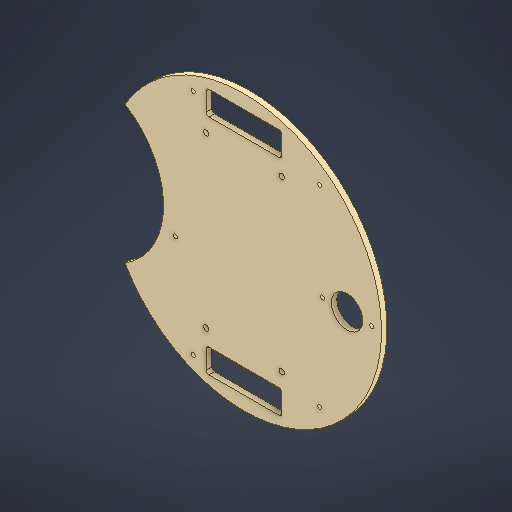
# Autodesk Inventor part: base plate
Saved by Autodesk Inventor 2026.1 (Build 301233000, 233)
## iProperties
Created: 2025-03-16
Part Number: base plate
Material: Generisch
Document SubType Name: Modeling
Designer: sfz
Density: 1 g/cm^3
Appearance: Beige
Author: sfz
Autodesk Inventor part; units mm, degrees
ref_plane "YZ Plane" through (0, 0, 0) normal (1, 0, 0) x (0, 1, 0)
ref_plane "XZ Plane" through (0, 0, 0) normal (0, 1, 0) x (-1, 0, 0)
ref_plane "XY Plane" through (0, 0, 0) normal (0, 0, 1) x (1, 0, 0)
sketch "Skizze1" plane through (0, 0, 0) normal (0, 1, 0) x (-1, 0, 0)
  arc A0 (86.6025, 50) -> (86.6025, -50) centre (0, 0) ccw
  arc A1 (86.6025, 50) -> (86.6025, -50) centre (117.2454, 0) ccw
  line L0 (27.5, 90) -> (-27.5, 90)
  line L1 (-27.5, 90) -> (-27.5, 72.5)
  line L2 (-27.5, 72.5) -> (27.5, 72.5)
  line L3 (27.5, 72.5) -> (27.5, 90)
  line L4 (27.5, -72.5) -> (-27.5, -72.5)
  line L5 (-27.5, -72.5) -> (-27.5, -90)
  line L6 (-27.5, -90) -> (27.5, -90)
  line L7 (27.5, -90) -> (27.5, -72.5)
  circle A2 centre (91, 0) radius 32
  circle A3 centre (27.5, 61.5) radius 2
  circle A4 centre (-27.5, 61.5) radius 2
  circle A5 centre (27.5, -61.5) radius 2
  circle A6 centre (-27.5, -61.5) radius 2
  circle A7 centre (-75, 0) radius 11.5
  circle A8 centre (-57, 0) radius 1.5
  circle A9 centre (-93, 0) radius 1.5
  circle A10 centre (50, -15) radius 1.5
  circle A11 centre (37, -83) radius 1.5
  circle A12 centre (37, 83) radius 1.5
  circle A13 centre (-55, 70) radius 1.5
  circle A14 centre (-55, -70) radius 1.5
  point P0 (58.6025, 0)
  point P1 (27.5, -81.25)
  dimension "d0" = 100
  dimension "d1" = 100
  dimension "d2" = 17.5
  dimension "d3" = 28
  dimension "d4" = 55
  dimension "d5" = 17.5
  dimension "d7" = 72.5
  dimension "d8" = 72.5
  dimension "d9" = 27.5
  dimension "d12" = 64
  dimension "d13" = 4
  dimension "d14" = 4
  dimension "d15" = 4
  dimension "d16" = 4
  dimension "d19" = 11
  dimension "d23" = 11
  dimension "d25" = 27.5
  dimension "d26" = 27.5
  dimension "d43" = 23
  dimension "d48" = 75
  dimension "d49" = 3
  dimension "d50" = 3
  dimension "d51" = 36
  dimension "d52" = 18
  dimension "d95" = 3
  dimension "d96" = 3
  dimension "d97" = 3
  dimension "d98" = 3
  dimension "d99" = 3
  dimension "d100" = 70
  dimension "d101" = 70
  dimension "d102" = 55
  dimension "d103" = 83
  dimension "d104" = 83
  dimension "d105" = 37
  dimension "d106" = 50
  dimension "d108" = 15
  constraints: 16 end point, 15 centre point, 6 horizontal alignment, 5 point on circle, 4 parallel, 4 vertical alignment, 2 horizontal, 2 perpendicular, 2 point on line, 1 coincident, 1 midpoint
  measures "d0" radius of A0
  measures "d1" distance of A1.start A1.end
  measures "d2" distance of L7.start L7.end
  measures "d3" horizontal distance of point (58.603, 0) A1.end
  measures "d4" distance from line of L5 point (27.5, -81.25)
  measures "d5" distance between parallel lines of L2 L0
  measures "d7" distance from line of L2 A0.centre
  measures "d8" distance from line of A0.centre L4
  measures "d9" distance from line of A0.centre L1
  measures "d12" diameter of A2
  measures "d13" diameter of A6
  measures "d14" diameter of A5
  measures "d15" diameter of A3
  measures "d16" diameter of A4
  measures "d19" distance from line of L4 A5.centre
  measures "d23" distance from line of L2 A3.centre
  measures "d25" horizontal distance of A0.centre A6.centre
  measures "d26" horizontal distance of A5.centre point (0, 0)
  measures "d43" diameter of A7
  measures "d48" distance of A0.centre A7.centre
  measures "d49" diameter of A8
  measures "d50" diameter of A9
  measures "d51" distance of A8.centre A9.centre
  measures "d52" distance of A9.centre A7.centre
  measures "d95" diameter of A11
  measures "d96" diameter of A14
  measures "d97" diameter of A13
  measures "d98" diameter of A12
  measures "d99" diameter of A10
  measures "d100" vertical distance of A0.centre A14.centre
  measures "d101" vertical distance of A13.centre A0.centre
  measures "d102" horizontal distance of A0.centre A14.centre
  measures "d103" vertical distance of A0.centre A12.centre
  measures "d104" vertical distance of A0.centre A11.centre
  measures "d105" horizontal distance of A0.centre A11.centre
  measures "d106" horizontal distance of point (0, 0) A10.centre
  measures "d108" vertical distance of A10.centre point (0, 0)
extrude "Extrusion1" add sketch "Skizze1" along normal blind 4 contours A1 A0
fillet "Rundung1" radius 2 8 edges at (-27.5, 2, 72.5) (-27.5, 2, 90) (27.5, 2, 90) (27.5, 2, 72.5) (-27.5, 2, -72.5) (27.5, 2, -72.5) (27.5, 2, -90) (-27.5, 2, -90)
equation "\"d26\" = d25"
